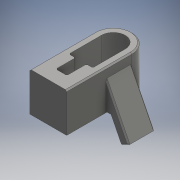
# Autodesk Inventor part: EndStopGeneric
Saved by Autodesk Inventor 2016 (Build 200138000, 138)
## iProperties
Created: 2016-10-31
Part Number: EndStopGeneric
Material: Generic
Document SubType Name: Modeling
Designer: mattc
Density: 1 g/cm^3
Appearance: Smooth - Medium Gray
Mass: 37.9952 g
Surface Area: 159.559 cm^2
Volume: 37.9952 cm^3
Author: mattc
Autodesk Inventor part; units mm, degrees
ref_plane "YZ Plane" through (0, 0, 0) normal (1, 0, 0) x (0, 1, 0)
ref_plane "XZ Plane" through (0, 0, 0) normal (0, 1, 0) x (-1, 0, 0)
sketch "Sketch1" plane through (0, 0, 0) normal (0, 0, 1) x (1, 0, 0)
  line L0 (-9.235, 1) -> (9.235, 1)
  line L1 (11.235, 1.1946) -> (11.235, -1)
  line L2 (11.235, -1) -> (-11.235, -1)
  line L3 (-11.235, -1) -> (-11.235, 1.0973)
  line L4 (-9.235, 1) -> (-9.235, 13.5)
  line L5 (-9.235, 13.5) -> (-11.235, 13.5)
  line L6 (-11.235, 13.5) -> (-11.235, 1.0973)
  line L7 (9.235, 1) -> (9.235, 13.5)
  line L8 (9.235, 13.5) -> (11.235, 13.5)
  line L9 (11.235, 13.5) -> (11.235, 1.1946)
  line L10 (-14.235, -4) -> (14.065, -4)
  line L11 (14.065, -4) -> (14.065, 46)
  line L12 (14.065, 46) -> (-14.235, 46)
  line L13 (-14.235, 46) -> (-14.235, -4)
  arc A0 (14.065, 46) -> (-14.235, 46) centre (-0.085, 46) ccw
  point P0 (0, 0)
  point P1 (0, 0)
  dimension "d0" = 22.47
  dimension "d1" = 11.235
  dimension "d3" = 1
  dimension "d4" = 14.5
  dimension "d5" = 2
  dimension "d6" = 2
  dimension "d7" = 14.5
  dimension "d10" = 2
  dimension "d19" = 28.3
  dimension "d20" = 50
  dimension "d21" = 14.15
  dimension "d22" = 3
  dimension "d23" = 3
  dimension "d64" = 18.47
  constraints: 28 end point, 6 parallel, 6 perpendicular, 2 horizontal, 2 point on circle, 1 centre point, 1 coincident
  measures "d0" distance of L1.end L2.end
  measures "d1" distance from line of L3 point (0, 0)
  measures "d3" distance from line of L2 point (0, 0)
  measures "d4" distance of L5.end L2.end
  measures "d5" distance of L4.end L5.end
  measures "d6" distance of L7.end L8.end
  measures "d7" distance of L1.end L8.end
  measures "d10" distance between parallel lines of L2 L0
  measures "d19" distance of L12.end L11.end
  measures "d20" distance of L11.end L10.end
  measures "d21" radius of A0
  measures "d22" distance between parallel lines of L10 L2
  measures "d23" distance between parallel lines of L6 L13
  measures "d64" distance of L0.start L0.end
extrude "Extrusion2" add sketch "Sketch1" along normal blind 25
sketch "Sketch2" plane through (0, 0, 25) normal (0, 0, 1) x (1, 0, 0)
  line L0 (-14.235, 46) -> (-14.235, -4) projected
  line L1 (-14.235, -4) -> (14.065, -4) projected
  line L2 (14.065, -4) -> (14.065, 46) projected
  line L3 (14.065, -4) -> (14.065, 46) projected
  line L4 (-14.235, -4) -> (14.065, -4)
  line L5 (14.065, -4) -> (14.065, 46)
  line L6 (-14.235, 46) -> (-14.235, -4)
  arc A0 (14.065, 46) -> (-14.235, 46) centre (-0.085, 46) ccw
  point P0 (0, 0)
  constraints: 6 end point, 2 point on circle, 2 tangent, 1 centre point, 1 horizontal, 1 parallel, 1 perpendicular
extrude "Extrusion3" add sketch "Sketch2" along normal blind 5
ref_plane "Work Plane1" through (-14.235, 46, 0) normal (0, -1, 0) x (1, 0, 0)
sketch "Sketch3" plane through (-14.235, 46, 0) normal (0, -1, 0) x (1, 0, 0)
  line L0 (0, 0) -> (28.3, 0) projected
  line L1 (28.3, 0) -> (28.3, 30) projected
  line L2 (0, 30) -> (28.3, 30) projected
  line L3 (0, 0) -> (0, 30) projected
  line L4 (14.235, 0) -> (42.81, 0) construction
  line L5 (28.3, 0) -> (28.3, 30) projected
  line L6 (31.8032, 0) -> (39.7036, -15.7866)
  line L7 (39.7036, -15.7866) -> (45.9635, -12.6539)
  line L8 (45.9635, -12.6539) -> (28.3, 22.6411)
  line L9 (28.3, 0) -> (0, 0) projected
  line L10 (28.3, 0) -> (31.8032, 0)
  line L11 (-3.5032, 0) -> (-11.4036, -15.7866)
  line L12 (-11.4036, -15.7866) -> (-17.6635, -12.6539)
  line L13 (-17.6635, -12.6539) -> (0, 22.6411)
  line L14 (0, 0) -> (-3.5032, 0)
  line L15 (0, 0) -> (0, 22.6411)
  dimension "d31" = 7
  constraints: 20 end point, 2 perpendicular, 2 point on line, 1 collinear, 1 horizontal
  measures "d31" distance of L6.end L7.end
extrude "Extrusion4" add sketch "Sketch3" along normal blind 20 contours L14 L11 L12 L13 L3 | L1 L8 L7 L6 L10
sketch "Sketch4" plane through (0, 0, 0) normal (0, 0, -1) x (-1, 0, 0)
  line L0 (14.235, -4) -> (-14.065, -4) projected
  line L1 (0.085, -4) -> (0.085, 46)
  arc A0 (9.235, 46) -> (-9.065, 46) centre (0.085, 46) ccw
  line L2 (-9.065, 46) -> (-9.065, 21)
  line L3 (9.235, 46) -> (9.235, 21)
  arc A1 (14.235, 46) -> (-14.065, 46) centre (0.085, 46) ccw projected
  line L4 (-4.235, 21) -> (-4.235, 6)
  line L5 (-4.235, 6) -> (4.235, 6)
  line L6 (4.235, 6) -> (4.235, 21)
  line L7 (11.235, 13.5) -> (9.235, 13.5) projected
  line L8 (9.235, 13.5) -> (9.235, 1) projected
  line L9 (9.235, 1) -> (-9.235, 1) projected
  line L10 (-9.235, 1) -> (-9.235, 13.5) projected
  line L11 (-9.235, 13.5) -> (-11.235, 13.5) projected
  line L12 (-11.235, 13.5) -> (-11.235, -1) projected
  line L13 (-11.235, -1) -> (11.235, -1) projected
  line L14 (11.235, -1) -> (11.235, 13.5) projected
  line L15 (-9.065, 21) -> (-4.235, 21)
  line L16 (4.235, 21) -> (9.235, 21)
  point P0 (0, 0)
  dimension "d34" = 50
  dimension "d38" = 25
  dimension "d46" = 5
  dimension "d47" = 5
  dimension "d48" = 5
  dimension "d49" = 5
  constraints: 16 end point, 4 perpendicular, 2 point on circle, 2 vertical, 1 centre point, 1 coincident, 1 midpoint, 1 parallel
  measures "d34" distance of L1.start L1.end
  measures "d38" distance of L2.start L2.end
  measures "d46" radial gap between concentric circles of A1 A0
  measures "d47" distance between parallel lines of L8 L6
  measures "d48" distance between parallel lines of L4 L10
  measures "d49" distance between parallel lines of L5 L9
extrude "Extrusion5" cut sketch "Sketch4" against normal blind 30 contours L5 L4 L15 L2 A0 L3 L16 L6
chamfer "Chamfer1" distance 1 angle 45 6 edges at (-4.235, 21, 15) (4.235, 21, 15) (-4.235, 6, 15) (4.235, 6, 15) (9.065, 21, 15) (-9.235, 21, 15)
chamfer "Chamfer3" distance 1 angle 45 8 edges at (22.8967, 26, 4.9936) (28.5986, 26, -14.2202) (21.5184, 26, -7.8933) (15.8166, 26, 0) (-15.9866, 26, 0) (-21.6884, 26, -7.8933) (-28.7686, 26, -14.2202) (-23.0667, 26, 4.9936)
chamfer "Chamfer4" distance 1 angle 45 8 edges at (15.8166, 46, 0) (21.5184, 46, -7.8933) (22.8967, 46, 4.9936) (28.5986, 46, -14.2202) (-23.0667, 46, 4.9936) (-28.7686, 46, -14.2202) (-15.9866, 46, 0) (-21.6884, 46, -7.8933)
chamfer "Chamfer5" distance 1 angle 45 3 edges at (-0.085, 60.15, 30) (-14.235, 21, 30) (14.065, 21, 30)
equation "\"d1\" = 0.5 * d0"
equation "\"d3\" = 0.5 * d10"
equation "\"d6\" = d5"
equation "\"d7\" = d4"
equation "\"d10\" = d5"
body "Solid2"
